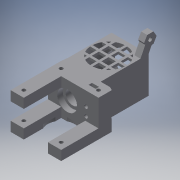
# Autodesk Inventor part: Extruder Body
Saved by Autodesk Inventor 2018 (Build 220112000, 112)
## iProperties
Created: 2018-05-13
Part Number: Extruder Body
Material: Generic
Document SubType Name: Modeling
Designer: Jasper
Density: 1 g/cm^3
Appearance: Default
Author: Jasper
Autodesk Inventor part; units mm, degrees
ref_plane "YZ Plane" through (0, 0, 0) normal (1, 0, 0) x (0, 1, 0)
ref_plane "XZ Plane" through (0, 0, 0) normal (0, 1, 0) x (-1, 0, 0)
ref_plane "XY Plane" through (0, 0, 0) normal (0, 0, 1) x (1, 0, 0)
sketch "Sketch2" plane through (0, 0, 0) normal (0, 0, 1) x (1, 0, 0)
  circle A0 centre (-1.7873, -12.6179) radius 1.5 projected
  circle A1 centre (-1.7873, 18.3821) radius 1.5 projected
  circle A2 centre (-32.7873, 18.3821) radius 1.5 projected
  line L0 (-1.7873, -12.6179) -> (-1.7873, 18.3821) construction
  line L1 (-1.7873, 18.3821) -> (-32.7873, 18.3821) construction
  line L2 (3.7127, -18.1179) -> (-7.2873, -18.1179)
  line L3 (-7.2873, -18.1179) -> (-7.2873, 23.8821)
  line L4 (-7.2873, 23.8821) -> (3.7127, 23.8821)
  line L5 (3.7127, 23.8821) -> (3.7127, -18.1179)
  line L6 (3.7127, -18.1179) -> (-7.2873, 23.8821) construction
  line L7 (-7.2873, -18.1179) -> (3.7127, 23.8821) construction
  line L8 (-38.2873, 12.8821) -> (3.7127, 12.8821)
  line L9 (3.7127, 12.8821) -> (3.7127, 23.8821)
  line L10 (3.7127, 23.8821) -> (-38.2873, 23.8821)
  line L11 (-38.2873, 23.8821) -> (-38.2873, 12.8821)
  line L12 (-38.2873, 12.8821) -> (3.7127, 23.8821) construction
  line L13 (3.7127, 12.8821) -> (-38.2873, 23.8821) construction
  circle A3 centre (-17.2873, 2.8821) radius 11
  line L14 (-9.9373, 32.2821) -> (-34.6373, 32.2821) construction
  line L15 (-9.9373, 63.8821) -> (-34.6373, 63.8821) construction
  line L16 (-9.9373, 32.2821) -> (-9.9373, 63.8821) construction
  line L17 (-34.6373, 63.8821) -> (-34.6373, 32.2821) construction
  line L18 (-37.6373, 29.2821) -> (-6.9373, 29.2821)
  line L19 (-6.9373, 29.2821) -> (-6.9373, 66.8821)
  line L20 (-6.9373, 66.8821) -> (-37.6373, 66.8821) construction
  line L21 (-37.6373, 66.8821) -> (-37.6373, 29.2821)
  line L22 (3.7127, 23.8821) -> (-6.9373, 29.2821)
  line L23 (-38.2873, 23.8821) -> (-37.6373, 29.2821)
  line L24 (-30.3873, 66.5821) -> (-14.1873, 66.5821) construction
  line L25 (-6.9373, 65.0821) -> (-37.6373, 65.0821)
  line L26 (3.7127, -12.2037) -> (3.7127, 17.9679) construction
  circle A4 centre (-32.7873, -12.6179) radius 1.5
  line L27 (-32.7873, -12.6179) -> (-32.7873, 18.3821) construction
  line L28 (-27.2873, -18.1179) -> (-38.2873, -18.1179)
  line L29 (-38.2873, -18.1179) -> (-38.2873, 23.8821)
  line L30 (-38.2873, 23.8821) -> (-27.2873, 23.8821)
  line L31 (-27.2873, 23.8821) -> (-27.2873, -18.1179)
  line L32 (-27.2873, -18.1179) -> (-38.2873, 23.8821) construction
  line L33 (-38.2873, -18.1179) -> (-27.2873, 23.8821) construction
  point P0 (0, 0)
  point P1 (-1.7873, 2.8821)
  point P2 (-17.2873, 18.3821)
  point P3 (-32.7873, 2.8821)
  dimension "d5" = 3
  dimension "d6" = 1.5
  constraints: 68 end point, 9 midpoint, 8 parallel, 6 horizontal, 6 perpendicular, 4 vertical, 2 centre point, 2 point on line, 1 collinear, 15 other
  measures "d5" distance between parallel lines of L14 L18
  measures "d6" distance between parallel lines of L25 L24
ref_plane "Work Plane3" through (-40.3873, -23.2104, 15) normal (0, 0, 1) x (1, 0, 0)
extrude "Extrusion1" add sketch "Sketch2" along normal up to surface (15 mm away) contours L2 L3 A3 L8 L5 | L8 L3 L4 L5 | L3 A3 | L4 L10 L23 L18 L22 | L8 A3 L31 L10 L3 | L31 L28 L29 L8 A3 | A3 L31 | L18 L21 L25 L19 | L8 A3 | L31 L8 L11 L10
sketch "Sketch4" plane through (-38.2873, 12.8821, 15) normal (0, 0, 1) x (1, 0, 0)
  line L0 (31.35, 52.2) -> (0.65, 52.2) construction
  line L1 (16, 52.2) -> (16, 0) construction
  line L2 (11, 0) -> (31, 0) construction
  line L3 (16, 0) -> (7, 0) construction
  line L4 (7.8, 0) -> (7.8, 4.55)
  line L5 (7.8, 4.55) -> (10.2, 4.55)
  line L6 (10.2, 4.55) -> (10.2, 10.4)
  line L7 (10.2, 10.4) -> (7.8, 10.4)
  line L8 (7.8, 10.4) -> (7.8, 19.2)
  line L9 (7.8, 19.2) -> (3.45, 19.2)
  line L10 (3.45, 19.2) -> (3.45, 52.2)
  line L11 (3.45, 52.2) -> (16, 52.2)
  line L12 (16, 52.2) -> (16, 0)
  line L13 (16, 0) -> (7.8, 0)
  line L14 (8, 4.75) -> (8, 1) construction
  line L15 (8, 4.75) -> (24, 4.75) construction
  line L16 (10, 10.2) -> (10, 4.75) construction
  line L17 (8, 10.2) -> (24, 10.2) construction
  line L18 (8, 13) -> (8, 10.2) construction
  line L19 (28.35, 19.4) -> (3.65, 19.4) construction
  line L20 (3.65, 19.4) -> (3.65, 20.85) construction
  point P0 (38.2873, -12.8821)
  point P1 (0, 0)
  dimension "d20" = 0.2
  dimension "d21" = 0.2
  dimension "d22" = 0.2
  dimension "d23" = 0.2
  dimension "d24" = 0.2
  dimension "d25" = 0.2
  dimension "d26" = 0.2
  constraints: 32 end point, 6 perpendicular, 6 vertical, 3 collinear, 3 point on line, 1 horizontal, 1 midpoint, 7 other
  measures "d20" distance between parallel lines of L4 L14
  measures "d21" distance between parallel lines of L15 L5
  measures "d22" distance between parallel lines of L16 L6
  measures "d23" distance between parallel lines of L7 L17
  measures "d24" distance between parallel lines of L18 L8
  measures "d25" distance between parallel lines of L19 L9
  measures "d26" distance between parallel lines of L20 L10
revolve "Revolution1" cut sketch "Sketch4" angle 360 about axis through (-22.2873, 65.0821, 15) along (0, -1, 0)
mirror "Mirror1" about plane through (-17.2873, 23.4821, 15) normal (0, 0, 1) of "Extrusion1", "Revolution1"
sketch "Sketch5" plane through (0, 0, 0) normal (0, 0, -1) x (-1, 0, 0)
  circle A0 centre (34.2873, 35.2821) radius 1.75 construction
  circle A1 centre (10.2873, 35.2821) radius 1.75 construction
  circle A2 centre (10.2873, 59.2821) radius 1.75 construction
  circle A3 centre (34.2873, 59.2821) radius 1.75 construction
  circle A4 centre (34.2873, 35.2821) radius 1.5
  circle A5 centre (10.2873, 35.2821) radius 1.5
  circle A6 centre (34.2873, 59.2821) radius 1.5
  circle A7 centre (10.2873, 59.2821) radius 1.5
  point P0 (0, 0)
  dimension "d27" = 3
  constraints: 4 centre point, 4 coincident, 3 equal radius
  measures "d27" diameter of A4
extrude "Extrusion2" cut sketch "Sketch5" against normal blind 6
sketch "Sketch6" plane through (0, 0, 0) normal (0, 0, -1) x (-1, 0, 0)
  circle A0 centre (22.2873, 47.2821) radius 14.375 projected
  point P0 (0, 0)
extrude "Extrusion3" cut sketch "Sketch6" against normal through all
sketch "Sketch7" plane through (-38.2873, 12.8821, 30) normal (0, 0, 1) x (1, 0, 0)
  circle A0 centre (16, 34.4) radius 14.375 construction
  line L0 (16, 20.025) -> (16, 48.775) construction
  line L1 (30.375, 34.4) -> (1.625, 34.4) construction
  line L2 (8, 20.025) -> (8, 48.775) construction
  line L3 (30.375, 42.4) -> (1.625, 42.4) construction
  line L4 (24, 20.025) -> (24, 48.775) construction
  line L5 (30.375, 26.4) -> (1.625, 26.4) construction
  line L6 (17, 48.775) -> (15, 48.775)
  line L7 (15, 48.775) -> (15, 20.025)
  line L8 (15, 20.025) -> (17, 20.025)
  line L9 (17, 20.025) -> (17, 48.775)
  line L10 (17, 48.775) -> (15, 20.025) construction
  line L11 (15, 48.775) -> (17, 20.025) construction
  line L12 (9, 46.9555) -> (7, 46.9555)
  line L13 (7, 46.9555) -> (7, 21.8445)
  line L14 (7, 21.8445) -> (9, 21.8445)
  line L15 (9, 21.8445) -> (9, 46.9555)
  line L16 (9, 46.9555) -> (7, 21.8445) construction
  line L17 (7, 46.9555) -> (9, 21.8445) construction
  line L18 (30.375, 33.4) -> (1.625, 33.4)
  line L19 (1.625, 33.4) -> (1.625, 35.4)
  line L20 (1.625, 35.4) -> (30.375, 35.4)
  line L21 (30.375, 35.4) -> (30.375, 33.4)
  line L22 (30.375, 33.4) -> (1.625, 35.4) construction
  line L23 (1.625, 33.4) -> (30.375, 35.4) construction
  circle A1 centre (16, 34.4) radius 14.375
  circle A2 centre (16, 34.4) radius 14.375 projected
  line L24 (31.35, 52.2) -> (0.65, 52.2) construction
  line L25 (16, 52.2) -> (16, 48.775) construction
  line L26 (28.5555, 41.4) -> (3.4445, 41.4)
  line L27 (3.4445, 41.4) -> (3.4445, 43.4)
  line L28 (3.4445, 43.4) -> (28.5555, 43.4)
  line L29 (28.5555, 43.4) -> (28.5555, 41.4)
  line L30 (28.5555, 41.4) -> (3.4445, 43.4) construction
  line L31 (3.4445, 41.4) -> (28.5555, 43.4) construction
  line L32 (23, 46.9555) -> (25, 46.9555)
  line L33 (25, 46.9555) -> (25, 21.8445)
  line L34 (25, 21.8445) -> (23, 21.8445)
  line L35 (23, 21.8445) -> (23, 46.9555)
  line L36 (28.5555, 27.4) -> (3.4445, 27.4)
  line L37 (3.4445, 27.4) -> (3.4445, 25.4)
  line L38 (3.4445, 25.4) -> (28.5555, 25.4)
  line L39 (28.5555, 25.4) -> (28.5555, 27.4)
  point P0 (38.2873, -12.8821)
  point P1 (8, 34.4)
  point P2 (16, 42.4)
  dimension "d34" = 8
  dimension "d41" = 8
  dimension "d46" = 2
  constraints: 78 end point, 13 midpoint, 12 symmetric about line, 8 parallel, 6 horizontal, 6 point on circle, 5 perpendicular, 4 equal length, 2 vertical, 1 centre point, 1 coincident, 1 concentric, 1 tangent, 6 other
  measures "d34" distance of L0.start L2.start
  measures "d41" distance of L1.start L3.start
  measures "d46" distance between parallel lines of L9 L7
extrude "Extrusion4" add sketch "Sketch7" against normal blind 2 contours L9 A1 L6 | A1 L7 L6 | A1 L9 L28 L7 | L28 L35 L26 L9 | L9 L26 L7 L28 | L32 L33 A1 | A1 L33 L28 L35 | L7 L26 L15 L28 | A1 L13 L12 | L15 L28 L13 A1 | L9 L20 L7 L26 | L28 L33 L26 L35 | L15 L26 L13 L28 | L20 L35 L18 L9 | L9 L18 L7 L20 | L26 L33 L20 L35 | L28 A1 L26 L33 | L28 L29 A1 | L7 L18 L15 L20 | L15 L20 L13 L26 | L13 L26 A1 L28 | A1 L27 L28 | L9 L36 L7 L18 | L20 L33 L18 L35 | L15 L18 L13 L20 | L36 L35 L38 L9 | L9 L38 L7 L36 | L18 L33 L36 L35 | L20 A1 L18 L33 | L20 L21 A1 | L7 L38 L15 L36 | L15 L36 L13 L18 | L13 L18 A1 L20 | A1 L19 L20 | L9 A1 L7 L38 | L36 L33 L38 L35 | L21 L18 A1 | L15 L38 L13 L36 | A1 L18 L19 | L9 L8 A1 | L38 L33 A1 L35 | L36 A1 L38 L33 | A1 L8 L7 | L15 A1 L13 L38 | L13 L38 A1 L36 | A1 L33 L34 | L39 L38 A1 | L14 L13 A1 | A1 L38 L37
sketch "Sketch8" plane through (-38.2873, 12.8821, 30) normal (0, 0, 1) x (1, 0, 0)
  line L0 (11, 0) -> (31, 0) projected
  line L1 (42, -31) -> (31, -31)
  line L2 (31, -31) -> (31, 0)
  line L3 (31, 0) -> (42, 0)
  line L4 (42, 0) -> (42, -31)
  point P0 (38.2873, -12.8821)
  point P1 (0, 0)
  constraints: 8 end point, 2 parallel, 1 horizontal, 1 perpendicular
extrude "Extrusion5" cut sketch "Sketch8" against normal blind 22
sketch "Sketch10" plane through (-38.2873, 12.8821, 0) normal (0, -1, 0) x (1, 0, 0)
  line L0 (42, 8) -> (31, 8) construction
  line L1 (31, 0) -> (31, 8) construction
  line L2 (31, 0) -> (42, 0) construction
  line L3 (42, 0) -> (42, 8) construction
  line L4 (38, 8) -> (35, 8) construction
  line L5 (38, 0) -> (35, 0) construction
  line L6 (38, 30) -> (35, 30) construction
  line L7 (-10.6712, 15) -> (50.7785, 15) construction
  line L8 (35, 30) -> (35, 8) construction
  line L9 (11, 30) -> (42, 30) construction
  line L10 (31.5, 30) -> (31.5, 8) construction
  circle A0 centre (31.5, 11.5) radius 1.6
  point P0 (38.2873, 0)
  point P1 (0, 30)
  dimension "d55" = 3.5
  dimension "d56" = 3.2
  dimension "d57" = 3.5
  constraints: 6 end point, 2 perpendicular, 2 point on line, 1 centre point, 1 horizontal, 2 other
  measures "d55" distance between parallel lines of L8 L10
  measures "d56" diameter of A0
  measures "d57" distance from line of L7 A0.centre
extrude "Extrusion6" cut sketch "Sketch10" against normal blind 8
sketch "Sketch11" plane through (-6.7873, 20.8821, 11.5) normal (0, -1, 0) x (1, 0, 0)
  line L0 (0, -3.3486) -> (-2.9, -1.6743)
  line L1 (-2.9, -1.6743) -> (-2.9, 1.6743)
  line L2 (-2.9, 1.6743) -> (0, 3.3486)
  line L3 (0, 3.3486) -> (2.9, 1.6743)
  line L4 (2.9, 1.6743) -> (2.9, -1.6743)
  line L5 (2.9, -1.6743) -> (0, -3.3486)
  circle A0 centre (0, 0) radius 1.6 construction
  line L6 (2.9, -1.6743) -> (-2.9, -1.6743)
  line L7 (-2.9, -1.6743) -> (-2.9, -11.5)
  line L8 (-2.9, -11.5) -> (2.9, -11.5)
  line L9 (2.9, -11.5) -> (2.9, -1.6743)
  line L10 (-25.5858, -11.5) -> (4.5858, -11.5) construction
  point P0 (6.7873, -11.5)
  dimension "d60" = 5.8
  constraints: 20 end point, 2 collinear, 2 parallel, 1 coincident, 1 horizontal, 1 perpendicular, 1 vertical, 13 other
  measures "d60" distance between parallel lines of L1 L4
extrude "Extrusion7" cut sketch "Sketch11" along normal blind 2.8
mirror "Mirror2" about plane through (-40.3873, -23.2104, 15) normal (0, 0, 1) of "Extrusion6", "Extrusion7"
sketch "Sketch12" plane through (-7.2873, -18.1179, 0) normal (0, -1, 0) x (1, 0, 0)
  circle A0 centre (0.5, 11.5) radius 1.6 construction
  circle A1 centre (0.5, 11.5) radius 1.6 projected
  circle A2 centre (0.5, 11.5) radius 3.5
  line L0 (7, 8) -> (4, 8) construction
  line L1 (7, 0) -> (4, 0) construction
  line L2 (4, 0) -> (4, 8) construction
  line L3 (11, 0) -> (0.35, 0) construction
  point P0 (7.2873, 0)
  constraints: 2 end point, 1 centre point, 1 coincident, 1 perpendicular, 1 tangent
extrude "Extrusion8" cut sketch "Sketch12" against normal up to surface (31 mm away) contours A1 | A2
sketch "Sketch14" plane through (-27.2873, -18.1179, 0) normal (1, 0, 0) x (0, 0, -1)
  line L0 (-8, 31) -> (-8, 0) projected
  line L1 (-15, -20.37) -> (-15, 122.22) construction
  line L2 (-22, 31) -> (-22, 0)
  line L3 (-8, 0) -> (-22, 0)
  line L4 (0, 0) -> (-30, 0) projected
  line L5 (-8, 31) -> (-22, 31)
  line L6 (0, 35) -> (-30, 35) projected
  point P0 (0, 18.1179)
  constraints: 8 end point, 2 symmetric about line, 1 collinear, 1 parallel, 1 vertical, 2 other
extrude "Extrusion9" cut sketch "Sketch14" against normal through all
sketch "Sketch15" plane through (0, 0, 0) normal (0, 0, -1) x (-1, 0, 0)
  circle A0 centre (17.2873, 2.8821) radius 11 construction
  circle A1 centre (17.2873, 2.8821) radius 11.2
  point P0 (0, 0)
  dimension "d68" = 0.2
  constraints: 1 centre point, 1 coincident
  measures "d68" radial gap between concentric circles of A0 A1
extrude "Extrusion10" cut sketch "Sketch15" against normal blind 3
sketch "Sketch16" plane through (3.7127, -18.1179, 0) normal (1, 0, 0) x (0, 0, -1)
  line L0 (-30, 42) -> (0, 42) construction
  line L1 (-15, -20.37) -> (-15, 122.22) construction
  arc A0 (1.0647, 44.194) -> (5.4353, 49.1396) centre (3.25, 46.6668) ccw construction
  arc A1 (1.0647, 44.194) -> (5.4353, 49.1396) centre (3.25, 46.6668) ccw construction
  line L2 (5.4353, 49.1396) -> (3.4569, 50.8879) construction
  arc A2 (3.2928, 52.2006) -> (3.4569, 50.8879) centre (4.1191, 51.6372) ccw construction
  arc A3 (3.2928, 52.2006) -> (7.75, 66.6668) centre (-17.9, 66.65) ccw construction
  line L3 (7.75, 66.6668) -> (7.75, 92.0668) construction
  line L4 (7.75, 92.0668) -> (-12.25, 92.0668) construction
  line L5 (-12.25, 92.0668) -> (-12.25, 89.6227) construction
  arc A4 (-14.851, 87.7151) -> (-12.25, 89.6227) centre (-14.25, 89.6227) ccw construction
  arc A5 (-14.851, 87.7151) -> (-33.902, 84.908) centre (-21.4819, 66.6668) ccw construction
  arc A6 (-35.127, 84.9853) -> (-33.902, 84.908) centre (-34.4648, 85.7346) ccw construction
  line L6 (-35.127, 84.9853) -> (-37.5647, 87.1396) construction
  arc A7 (-37.5647, 87.1396) -> (-41.9353, 82.194) centre (-39.75, 84.6668) ccw construction
  line L7 (-41.9353, 82.194) -> (-39.8937, 80.3899) construction
  arc A8 (-39.7291, 79.0781) -> (-39.8937, 80.3899) centre (-40.5559, 79.6406) ccw construction
  arc A9 (-39.7291, 79.0781) -> (-43.55, 66.6668) centre (-21.4819, 66.6668) ccw construction
  arc A10 (-43.55, 66.6668) -> (-2.4169, 46.2001) centre (-17.9, 66.65) ccw construction
  arc A11 (-1.1511, 46.1522) -> (-2.4169, 46.2001) centre (-1.8133, 45.4029) ccw construction
  line L8 (-1.1511, 46.1522) -> (1.0647, 44.194) construction
  circle A12 centre (-19.75, 66.6668) radius 16 construction
  circle A13 centre (-39.75, 84.6668) radius 2.25 construction
  circle A14 centre (3.25, 46.6668) radius 2.25 construction
  arc A15 (-44.05, 66.667) -> (-2.1151, 45.8015) centre (-17.9, 66.65) ccw
  arc A16 (-40.1425, 79.3593) -> (-44.05, 66.667) centre (-21.4819, 66.6668) ccw
  arc A17 (-40.1425, 79.3593) -> (-40.2248, 80.0152) centre (-40.5559, 79.6406) ccw
  line L9 (-40.2248, 80.0152) -> (-42.2664, 81.8194)
  arc A18 (-37.2336, 87.5143) -> (-42.2664, 81.8194) centre (-39.75, 84.6668) ccw
  line L10 (-37.2336, 87.5143) -> (-34.7959, 85.3599)
  arc A19 (-34.7959, 85.3599) -> (-34.1834, 85.3213) centre (-34.4648, 85.7346) ccw
  arc A20 (-14.7007, 88.192) -> (-34.1834, 85.3213) centre (-21.4819, 66.6668) ccw
  arc A21 (-14.7007, 88.192) -> (-12.75, 89.6227) centre (-14.25, 89.6227) ccw
  line L11 (-12.75, 89.6227) -> (-12.75, 92.5668)
  line L12 (-12.75, 92.5668) -> (8.25, 92.5668)
  line L13 (8.25, 92.5668) -> (8.25, 66.65)
  arc A22 (3.706, 51.9189) -> (8.25, 66.65) centre (-17.9, 66.65) ccw
  arc A23 (3.706, 51.9189) -> (3.788, 51.2626) centre (4.1191, 51.6372) ccw
  line L14 (3.788, 51.2626) -> (5.7664, 49.5143)
  arc A24 (0.7336, 43.8194) -> (5.7664, 49.5143) centre (3.25, 46.6668) ccw
  line L15 (0.7336, 43.8194) -> (-1.4822, 45.7775)
  arc A25 (-1.4822, 45.7775) -> (-2.1151, 45.8015) centre (-1.8133, 45.4029) ccw
  point P0 (0, 18.1179)
  dimension "d74" = 0.5
  constraints: 22 point on circle, 16 end point, 11 centre point, 1 vertical, 19 other
  measures "d74" radial gap between concentric circles of A10 A15
extrude "Extrusion11" cut sketch "Sketch16" against normal up to surface (10.65 mm away)
sketch "Sketch17" plane through (0, 0, 0) normal (0, 0, -1) x (-1, 0, 0)
  line L0 (7.2873, 34.7821) -> (7.2873, 59.7821) construction
  arc A0 (7.2873, 34.7821) -> (9.7873, 32.2821) centre (9.7873, 34.7821) ccw construction
  line L1 (9.7873, 32.2821) -> (34.7873, 32.2821) construction
  arc A1 (34.7873, 32.2821) -> (37.2873, 34.7821) centre (34.7873, 34.7821) ccw construction
  line L2 (37.2873, 34.7821) -> (37.2873, 59.7821) construction
  arc A2 (37.2873, 59.7821) -> (34.7873, 62.2821) centre (34.7873, 59.7821) ccw construction
  line L3 (9.7873, 62.2821) -> (34.7873, 62.2821) construction
  arc A3 (9.7873, 62.2821) -> (7.2873, 59.7821) centre (9.7873, 59.7821) ccw construction
  circle A4 centre (22.2873, 47.2821) radius 14.375 construction
  circle A5 centre (34.2873, 35.2821) radius 1.75 construction
  circle A6 centre (10.2873, 35.2821) radius 1.75 construction
  circle A7 centre (34.2873, 59.2821) radius 1.75 construction
  circle A8 centre (10.2873, 59.2821) radius 1.75 construction
  line L4 (32.3731, 23.8821) -> (2.2015, 23.8821) construction
  line L5 (6.9373, 65.0821) -> (6.9373, 26.3498) construction
  line L6 (16.9373, 24.3821) -> (6.9373, 24.3821)
  line L7 (6.9373, 24.3821) -> (6.9373, 31.7821)
  line L8 (6.9373, 31.7821) -> (16.9373, 31.7821)
  line L9 (16.9373, 31.7821) -> (16.9373, 24.3821)
  point P0 (0, 0)
  dimension "d75" = 0.5
  dimension "d76" = 0.5
  dimension "d77" = 10
  constraints: 8 end point, 2 parallel, 1 collinear, 1 horizontal, 1 perpendicular
  measures "d75" distance between parallel lines of L1 L8
  measures "d76" distance between parallel lines of L4 L6
  measures "d77" distance of L7.end L8.end
extrude "Extrusion12" add sketch "Sketch17" along normal blind 8
sketch "Sketch18" plane through (-6.9373, 65.0821, 30) normal (1, 0, 0) x (0, 0, -1)
  circle A0 centre (33.25, -36.5332) radius 2.25 construction
  circle A1 centre (33.25, -36.5332) radius 1.6
  point P0 (30, -65.0821)
  dimension "d80" = 3.2
  constraints: 1 centre point, 1 coincident
  measures "d80" diameter of A1
extrude "Extrusion13" cut sketch "Sketch18" against normal through all
sketch "Sketch19" plane through (-16.9373, 24.3821, 0) normal (-1, 0, 0) x (0, 0, 1)
  circle A0 centre (-3.25, 4.1668) radius 1.6 construction
  line L0 (-3.25, 0.5295) -> (-6.4, 2.3481)
  line L1 (-6.4, 2.3481) -> (-6.4, 5.9855)
  line L2 (-6.4, 5.9855) -> (-3.25, 7.8041)
  line L3 (-3.25, 7.8041) -> (-0.1, 5.9855)
  line L4 (-0.1, 5.9855) -> (-0.1, 2.3481)
  line L5 (-0.1, 2.3481) -> (-3.25, 0.5295)
  point P0 (0, -24.3821)
  dimension "d83" = 6.3
  constraints: 12 end point, 1 coincident, 1 vertical, 13 other
  measures "d83" distance between parallel lines of L4 L1
extrude "Extrusion14" cut sketch "Sketch19" against normal blind 3.2
sketch "Sketch20" plane through (-6.9373, 65.0821, 30) normal (1, 0, 0) x (0, 0, -1)
  circle A0 centre (-9.75, 1.4668) radius 2.25 construction
  line L0 (-9.75, 1.4668) -> (0, -3.3455) construction
  line L1 (0, -39.7322) -> (0, 0) construction
  line L2 (-11.0778, -1.2234) -> (0, -6.691)
  line L3 (-8.4222, 4.157) -> (0, 0)
  circle A1 centre (-9.75, 1.4668) radius 3
  line L4 (-9.75, -3.7294) -> (-14.25, -1.1313)
  line L5 (-14.25, -1.1313) -> (-14.25, 4.0649)
  line L6 (-14.25, 4.0649) -> (-9.75, 6.663)
  line L7 (-9.75, 6.663) -> (-5.25, 4.0649)
  line L8 (-5.25, 4.0649) -> (-5.25, -1.1313)
  line L9 (-5.25, -1.1313) -> (-9.75, -3.7294)
  line L10 (0, 0) -> (0, -6.691)
  line L11 (30, 0) -> (0, 0) projected
  point P0 (30, -65.0821)
  dimension "d86" = 6
  dimension "d87" = 9
  constraints: 20 end point, 2 coincident, 2 point on circle, 2 point on line, 1 centre point, 1 parallel, 1 perpendicular, 1 tangent, 1 vertical, 14 other
  measures "d86" distance between parallel lines of L3 L2
  measures "d87" distance between parallel lines of L5 L8
extrude "Extrusion15" add sketch "Sketch20" against normal blind 5
sketch "Sketch21" plane through (-6.9373, 31.7821, 0) normal (1, 0, 0) x (0, 0, -1)
  line L0 (-39.75, 29.5706) -> (-44.25, 32.1687) construction
  line L1 (-39.75, 29.5706) -> (-39.75, 39.963) construction
  circle A0 centre (-39.75, 34.7668) radius 1.6
  line L2 (-44.25, 37.3649) -> (-39.75, 39.963) projected
  point P0 (0, -31.7821)
  dimension "d90" = 3.2
  constraints: 2 end point, 1 centre point, 1 midpoint, 1 point on line, 1 vertical
  measures "d90" diameter of A0
extrude "Extrusion16" cut sketch "Sketch21" against normal through all
sketch "Sketch22" plane through (-11.9373, 65.0821, 30) normal (-1, 0, 0) x (0, 0, 1)
  circle A0 centre (9.75, 1.4668) radius 1.6 construction
  line L0 (9.75, -2.1128) -> (6.65, -0.323)
  line L1 (6.65, -0.323) -> (6.65, 3.2566)
  line L2 (6.65, 3.2566) -> (9.75, 5.0464)
  line L3 (9.75, 5.0464) -> (12.85, 3.2566)
  line L4 (12.85, 3.2566) -> (12.85, -0.323)
  line L5 (12.85, -0.323) -> (9.75, -2.1128)
  point P0 (-30, -65.0821)
  dimension "d93" = 6.2
  constraints: 12 end point, 1 coincident, 1 vertical, 13 other
  measures "d93" distance between parallel lines of L1 L4
extrude "Extrusion17" cut sketch "Sketch22" against normal blind 3.2
body "Solid1"
